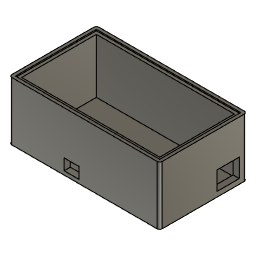
Box_v3 (Autodesk Fusion 360 design; units mm, degrees)
Autodesk Fusion 360 part; units mm, degrees
note: some values were not read from the file. Set by a fixed rule: which sketch regions a step uses.
sketch "Esquisse1" plane through (0, 0, 0) normal (0, 0, 1) x (1, 0, 0)
  line L0 (74.4967, -39.3812) -> (-42.7033, -39.3812)
  line L1 (-42.7033, 30.8188) -> (74.4967, 30.8188)
  line L2 (76.4967, 28.8188) -> (76.4967, -37.3812)
  line L3 (-44.7033, -37.3812) -> (-44.7033, 28.8188)
  arc A0 (76.4967, 28.8188) -> (74.4967, 30.8188) centre (74.4967, 28.8188) ccw
  arc A1 (-42.7033, 30.8188) -> (-44.7033, 28.8188) centre (-42.7033, 28.8188) ccw
  arc A2 (-44.7033, -37.3812) -> (-42.7033, -39.3812) centre (-42.7033, -37.3812) ccw
  arc A3 (74.4967, -39.3812) -> (76.4967, -37.3812) centre (74.4967, -37.3812) ccw
  point P0 (-37.2797, 0.2421)
  point P1 (-65.57, -27.6552)
  dimension "d25" = 121.2
  dimension "d26" = 70.2
  dimension "d31" = 2
  dimension "d32" = 2
  dimension "d33" = 2
  dimension "d34" = 2
  constraint horizontal L1
  constraint vertical L2
  constraint horizontal L0
  constraint vertical L3
  constraint tangent L1 A0
  constraint tangent L2 A0
  constraint tangent L3 A1
  constraint tangent L1 A1
  constraint tangent L3 A2
  constraint tangent L0 A2
  constraint tangent L0 A3
  constraint tangent L2 A3
  measures "d25" distance of L2 L3
  measures "d26" distance of L0 L1
  measures "d31" radius of A0
  measures "d32" radius of A1
  measures "d33" radius of A2
  measures "d34" radius of A3
extrude "Extrusion1" add sketch "Esquisse1" along normal blind 47
sketch "Esquisse2" plane through (0, 0, 47) normal (0, 0, 1) x (-1, 0, 0)
  arc A0 (44.7033, 37.3812) -> (42.7033, 39.3812) centre (42.7033, 37.3812) ccw
  line L0 (42.7033, 39.3812) -> (-74.4967, 39.3812)
  arc A1 (-74.4967, 39.3812) -> (-76.4967, 37.3812) centre (-74.4967, 37.3812) ccw
  line L1 (-76.4967, 37.3812) -> (-76.4967, -28.8188)
  arc A2 (-76.4967, -28.8188) -> (-74.4967, -30.8188) centre (-74.4967, -28.8188) ccw
  line L2 (-74.4967, -30.8188) -> (42.7033, -30.8188)
  arc A3 (42.7033, -30.8188) -> (44.7033, -28.8188) centre (42.7033, -28.8188) ccw
  line L3 (44.7033, -28.8188) -> (44.7033, 37.3812)
  line L4 (39.7033, -25.8188) -> (39.7033, 34.3812)
  line L5 (39.7033, 34.3812) -> (-71.4967, 34.3812)
  line L6 (-71.4967, 34.3812) -> (-71.4967, -25.8188)
  line L7 (-71.4967, -25.8188) -> (39.7033, -25.8188)
  line L8 (42.2033, -28.3188) -> (42.2033, 36.8812)
  line L9 (42.2033, 36.8812) -> (-73.9967, 36.8812)
  line L10 (-73.9967, 36.8812) -> (-73.9967, -28.3188)
  line L11 (-73.9967, -28.3188) -> (42.2033, -28.3188)
  dimension "d37" = -2.5
  dimension "d49" = -5
extrude "Extrusion2" cut sketch "Esquisse2" against normal blind 1 contours L4 L5 L6 L7 | L8 L9 L10 L11
extrude "Extrusion4" cut sketch "Esquisse2" against normal blind 45 contours L4 L5 L6 L7
sketch "Esquisse3" plane through (76.4967, 0, 0) normal (1, 0, 0) x (0, 1, 0)
  line L0 (-37.3812, 0) -> (28.8188, 0)
  line L1 (28.8188, 0) -> (28.8188, 47)
  line L2 (28.8188, 47) -> (-37.3812, 47)
  line L3 (-37.3812, 47) -> (-37.3812, 0)
  line L4 (6.8188, 19) -> (24.8188, 19)
  line L5 (24.8188, 19) -> (24.8188, 4)
  line L6 (24.8188, 4) -> (6.8188, 4)
  line L7 (6.8188, 4) -> (6.8188, 19)
  dimension "d40" = 18
  dimension "d42" = 19
  dimension "d44" = 4
  dimension "d47" = 15
  constraint horizontal L4
  constraint vertical L5
  constraint horizontal L6
  constraint vertical L7
  measures "d40" distance of L4.start L4.end
  measures "d42" distance of L0 L4
  measures "d44" distance of L1 L5
  measures "d47" distance of L4 L6
extrude "Extrusion3" cut sketch "Esquisse3" against normal blind 50 contours L4 L5 L6 L7
sketch "Esquisse4" plane through (0, -39.3812, 0) normal (0, -1, 0) x (1, 0, 0)
  line L0 (-42.7033, 0) -> (74.4967, 0)
  line L1 (74.4967, 0) -> (74.4967, 47)
  line L2 (74.4967, 47) -> (-42.7033, 47)
  line L3 (-42.7033, 47) -> (-42.7033, 0)
  line L4 (-0.5033, 12) -> (11.4967, 12)
  line L5 (11.4967, 12) -> (11.4967, 3)
  line L6 (11.4967, 3) -> (-0.5033, 3)
  line L7 (-0.5033, 3) -> (-0.5033, 12)
  dimension "d52" = 12
  dimension "d53" = 9
  dimension "d54" = 75
  dimension "d55" = 3
  constraint horizontal L4
  constraint vertical L5
  constraint horizontal L6
  constraint vertical L7
  measures "d52" distance of L4.start L4.end
  measures "d53" distance of L4.start L6.end
  measures "d54" distance of L1 L7
  measures "d55" distance of L0 L6
extrude "Extrusion5" cut sketch "Esquisse4" against normal blind 25 contours L4 L5 L6 L7
